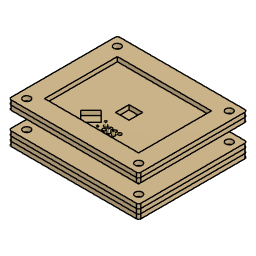
Solum Newton Lite 1.6 - Fusion360 (Autodesk Fusion 360 design; units mm, degrees)
Autodesk Fusion 360 part; units mm, degrees
sketch "Skizze1" plane through (0, 0, 0) normal (0, 0, 1) x (1, 0, 0)
  line L0 (21, -16.25) -> (-21, -16.25)
  line L1 (-21, -16.25) -> (-21, 16.25)
  line L2 (-21, 16.25) -> (21, 16.25)
  line L3 (21, 16.25) -> (21, -16.25)
  line L4 (21, -16.25) -> (-21, 16.25) construction
  line L5 (-21, -16.25) -> (21, 16.25) construction
  circle A0 centre (2.3, -12.95) radius 0.75
  circle A1 centre (3.3, -14.75) radius 0.45
  circle A2 centre (1.2, -11.15) radius 0.75
  circle A3 centre (7.5, -14.75) radius 0.45
  circle A4 centre (2.3, -12.95) radius 0.45
  circle A5 centre (3.3, -11.15) radius 0.75
  circle A6 centre (1.2, -14.75) radius 0.45
  circle A7 centre (4.4, -12.95) radius 0.75
  circle A8 centre (6.5, -12.95) radius 0.75
  circle A9 centre (5.4, -14.75) radius 0.45
  circle A10 centre (6.5, -12.95) radius 0.45
  circle A11 centre (1.2, -14.75) radius 0.75
  circle A12 centre (5.4, -14.75) radius 0.75
  circle A13 centre (7.5, -14.75) radius 0.75
  circle A14 centre (4.4, -12.95) radius 0.45
  circle A15 centre (7.5, -11.15) radius 0.45
  circle A16 centre (5.4, -11.15) radius 0.45
  circle A17 centre (3.3, -14.75) radius 0.75
  circle A18 centre (7.5, -11.15) radius 0.75
  circle A19 centre (3.3, -11.15) radius 0.45
  circle A20 centre (1.2, -11.15) radius 0.45
  circle A21 centre (5.4, -11.15) radius 0.75
  line L6 (28, -24.25) -> (-28, -24.25)
  line L7 (-29, -23.25) -> (-29, 23.25)
  line L8 (-28, 24.25) -> (28, 24.25)
  line L9 (29, 23.25) -> (29, -23.25)
  line L10 (-25, 20.25) -> (25, 20.25) construction
  line L11 (25, 20.25) -> (25, -20.25) construction
  line L12 (25, -20.25) -> (-25, -20.25) construction
  line L13 (-25, -20.25) -> (-25, 20.25) construction
  circle A22 centre (-25, 20.25) radius 1.6
  circle A23 centre (25, 20.25) radius 1.6
  circle A24 centre (25, -20.25) radius 1.6
  circle A25 centre (-25, -20.25) radius 1.6
  line L14 (-5.8, -15.3462) -> (-10.3962, -10.75)
  line L15 (-10.3962, -10.75) -> (-5.8, -6.1538)
  line L16 (-5.8, -6.1538) -> (-1.2038, -10.75)
  line L17 (-1.2038, -10.75) -> (-5.8, -15.3462)
  line L18 (-5.8, -15.3462) -> (-5.8, -6.1538) construction
  line L19 (-10.3962, -10.75) -> (-1.2038, -10.75) construction
  line L20 (4.2, -3.75) -> (-1.8, -3.75)
  line L21 (-1.8, -3.75) -> (-1.8, 2.25)
  line L22 (-1.8, 2.25) -> (4.2, 2.25)
  line L23 (4.2, 2.25) -> (4.2, -3.75)
  line L24 (4.2, -3.75) -> (-1.8, 2.25) construction
  line L25 (-1.8, -3.75) -> (4.2, 2.25) construction
  arc A26 (-28, 24.25) -> (-29, 23.25) centre (-28, 23.25) ccw
  arc A27 (29, 23.25) -> (28, 24.25) centre (28, 23.25) ccw
  arc A28 (-29, -23.25) -> (-28, -24.25) centre (-28, -23.25) ccw
  arc A29 (28, -24.25) -> (29, -23.25) centre (28, -23.25) ccw
  line L26 (9.4, -16.25) -> (-0.6, -16.25)
  line L27 (-0.6, -16.25) -> (-0.6, -10.65)
  line L28 (0.4, -9.65) -> (8.4, -9.65)
  line L29 (9.4, -10.65) -> (9.4, -16.25)
  line L30 (9.4, -16.25) -> (-0.6, -9.65) construction
  line L31 (-0.6, -16.25) -> (9.4, -9.65) construction
  arc A30 (0.4, -9.65) -> (-0.6, -10.65) centre (0.4, -10.65) ccw
  arc A31 (9.4, -10.65) -> (8.4, -9.65) centre (8.4, -10.65) ccw
  point P0 (4.3, -13.35)
  point P1 (4.3, -13.35)
  point P2 (-5.8, -10.75)
  point P3 (-5.8, -10.75)
  point P4 (1.2, -0.75)
  point P5 (1.2, -0.75)
  point P6 (4.4, -12.95)
  dimension "d1" = 42
  dimension "d2" = 32.5
  dimension "d5" = 1.5
  dimension "d6" = 0.9
  dimension "d9" = -4
  dimension "d10" = 3.2
  dimension "d11" = 6.5
  dimension "d12" = 6.5
  dimension "d13" = 6
  dimension "d14" = 6
  dimension "d19" = 1
  dimension "d20" = 1
  dimension "d21" = 1
  dimension "d22" = 1
  dimension "d23" = 10
  dimension "d30" = 1
  dimension "d31" = 1
  constraint horizontal L0
  constraint perpendicular L0 L1
  constraint parallel L0 L2
  constraint parallel L1 L3
  constraint coincident L4 origin
  constraint coincident L5 origin
  constraint coincident P1 P0
  constraint equal A2 A5
  constraint equal A2 A21
  constraint equal A2 A18
  constraint equal A2 A7
  constraint equal A2 A8
  constraint equal A2 A11
  constraint equal A2 A12
  constraint equal A2 A13
  constraint concentric A2 A20
  constraint concentric A5 A19
  constraint concentric A16 A21
  constraint concentric A15 A18
  constraint concentric A0 A4
  constraint concentric A7 A14
  constraint concentric A8 A10
  constraint concentric A6 A11
  constraint concentric A1 A17
  constraint concentric A9 A12
  constraint concentric A3 A13
  constraint equal A19 A20
  constraint equal A16 A20
  constraint equal A15 A20
  constraint equal A4 A20
  constraint equal A14 A20
  constraint equal A10 A20
  constraint equal A6 A20
  constraint equal A1 A20
  constraint equal A9 A20
  constraint equal A3 A20
  constraint coincident L10.start L13.end
  constraint coincident L10.end L11.start
  constraint coincident L11.end L12.start
  constraint coincident L12.end L13.start
  constraint equal A22 A23
  constraint equal A22 A25
  constraint equal A22 A24
  constraint perpendicular L14 L15
  constraint parallel L14 L16
  constraint parallel L15 L17
  constraint coincident L18 P3
  constraint coincident L19 P3
  constraint coincident P3 P2
  constraint horizontal L20
  constraint perpendicular L20 L21
  constraint parallel L20 L22
  constraint parallel L21 L23
  constraint coincident L24 P5
  constraint coincident L25 P5
  constraint coincident P5 P4
  constraint tangent L7 A26
  constraint tangent L8 A26
  constraint tangent L8 A27
  constraint tangent L9 A27
  constraint tangent L6 A28
  constraint tangent L7 A28
  constraint tangent L6 A29
  constraint tangent L9 A29
  constraint horizontal L26
  constraint perpendicular L26 L27
  constraint parallel L26 L28
  constraint parallel L27 L29
  constraint coincident L30 P6
  constraint coincident L31 P6
  constraint coincident P6 A7.centre
  constraint coincident L30.end L28
  constraint coincident L30.end L27
  constraint tangent L28 A30
  constraint tangent L27 A30
  constraint coincident L31.end L28
  constraint coincident L31.end L29
  constraint tangent L28 A31
  constraint tangent L29 A31
  measures "d1" distance of L1.end L2.end
  measures "d2" distance of L0.end L1.end
  measures "d5" diameter of A2
  measures "d6" diameter of A20
  measures "d10" diameter of A22
  measures "d11" distance of L15.end L16.end
  measures "d12" distance of L14.end L15.end
  measures "d13" distance of L21.end L22.end
  measures "d14" distance of L20.end L21.end
  measures "d19" radius of A26
  measures "d20" radius of A27
  measures "d21" radius of A28
  measures "d22" radius of A29
  measures "d23" distance of L30.end L31.end
  measures "d30" radius of A30
  measures "d31" radius of A31
extrude "Extrusion13" add sketch "Skizze1" along normal blind 2 contours L0 L1 L2 L3 L27 L28 L29 A30 A31 | L0 L26 L27 L28 L29 A30 A31 | A0 | A1 | A2 | A3 | A4 | A5 | A6 | A7 | A8 | A9 | A10 | A11 | A12 | A13 | A14 | A15 | A16 | A17 | A18 | A19 | A20 | A21 | L6 L7 L8 L9 A26 A27 A28 A29 | L14 L15 L16 L17 | L20 L21 L22 L23 makes body 1
extrude "Extrusion14" add sketch "Skizze1" along normal blind 2 separate body contours L0 L1 L2 L3 L27 L28 L29 A30 A31 | L0 L26 L27 L28 L29 A30 A31 | A0 | A2 | A5 | A7 | A8 | A11 | A12 | A13 | A17 | A18 | A21 | L6 L7 L8 L9 A26 A27 A28 A29 | L14 L15 L16 L17 | L20 L21 L22 L23 makes body 2
move_body "Verschieben2" bodies 2 to x (1, 0, 0) y (0, 1, 0) z (0, 0, 1) at (0, 0, 2)
extrude "Extrusion17" add sketch "Skizze1" along normal blind 2 separate body contours L0 L26 L27 L28 L29 A30 A31 | A0 | A2 | A5 | A7 | A8 | A11 | A12 | A13 | A17 | A18 | A21 | L6 L7 L8 L9 A26 A27 A28 A29 makes body 3
move_body "Verschieben5" bodies 3 to x (1, 0, 0) y (0, 1, 0) z (0, 0, 1) at (0, 0, 4)
extrude "Extrusion18" add sketch "Skizze1" along normal blind 2 separate body contours L0 L1 L2 L3 L27 L28 L29 A30 A31 | L0 L26 L27 L28 L29 A30 A31 | L6 L7 L8 L9 A26 A27 A28 A29 makes body 4
move_body "Verschieben6" bodies 4 to x (1, 0, 0) y (0, 1, 0) z (0, 0, 1) at (0, 0, 14)
extrude "Extrusion19" add sketch "Skizze1" along normal blind 2 separate body contours L6 L7 L8 L9 A26 A27 A28 A29 makes body 5
move_body "Verschieben7" bodies 5 to x (1, 0, 0) y (0, 1, 0) z (0, 0, 1) at (0, 0, 16)
extrude "Extrusion21" add sketch "Skizze1" along normal blind 16 separate body contours A6 | A10 | A14 | A20 makes body 6 at (1.6411, -11.2392, 10.6667) makes body 7 at (4.0858, -13.2721, 10.6667) makes body 8 at (1.6411, -14.8392, 10.6667) makes body 9 at (6.1858, -13.2721, 10.6667)
move_body "Verschieben9" bodies 6 9 8 7 to x (1, 0, 0) y (0, 1, 0) z (0, 0, 1) at (0, 0, 2)
chamfer "Fase2" distance 0.3 angle 45 4 faces at (1.3371, -11.3219, 18) (1.3371, -14.9219, 18) (4.5371, -13.1219, 18) (6.3632, -12.8626, 18) on bodies 6 7 8 9
named bodies: "Layer 0", "Layer 1", "Layer 2", "Layer 3", "Layer 4", "Pin VCC / ESP 16,17,18,21", "Pin CLK / ESP 33", "Pin GND / ESP GND", "Pin MISO / ESP 35"
